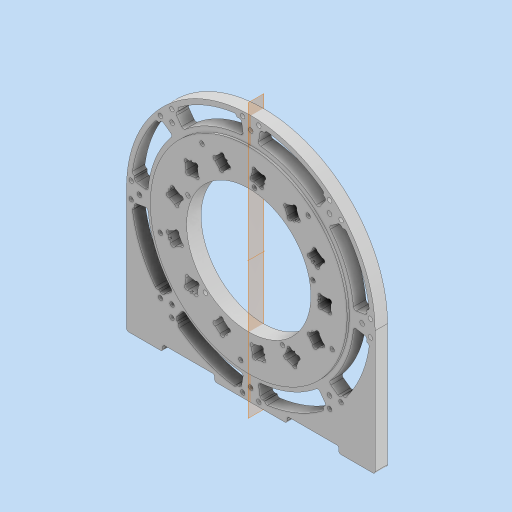
# Autodesk Inventor part: Ring_10_front
Saved by Autodesk Inventor 2024.2 (Build 282272000, 272)
## iProperties
Created: 2025-04-23
Part Number: Ring_10_front
Material: Generic
Document SubType Name: Modeling
Designer: 23661194
Density: 1 g/cm^3
Appearance: Default
Author: 23661194
Autodesk Inventor part; units mm, degrees
ref_plane "XZ Plane" through (0, 0, 0) normal (0, 1, 0) x (-1, 0, 0)
ref_plane "XY Plane" through (0, 0, 0) normal (0, 0, 1) x (1, 0, 0)
sketch "Shim Tray Slot" plane through (0, 0, 0) normal (0, 0, 1) x (1, 0, 0)
  line L0 (30.092, 109.0254) -> (29.9458, 108.3375)
  line L1 (33.5758, 105.3229) -> (31.6829, 97.1237)
  line L2 (-33.5758, 105.3229) -> (-31.6821, 97.1202)
  line L3 (-30.092, 109.0254) -> (-29.9458, 108.3375)
  arc A0 (-32.2001, 107.689) -> (-33.5758, 105.3229) centre (-31.6271, 105.7728) ccw
  arc A1 (29.147, 95.658) -> (-29.1504, 95.657) centre (0, 0) ccw
  arc A2 (28.6337, 111.3782) -> (-28.6337, 111.3782) centre (0, 0) ccw
  arc A3 (-29.9458, 108.3375) -> (-32.2001, 107.689) centre (0, 0) ccw
  arc A4 (32.2001, 107.689) -> (29.9458, 108.3375) centre (0, 0) ccw
  arc A5 (-28.6337, 111.3782) -> (-30.092, 109.0254) centre (-28.1357, 109.4412) ccw
  arc A6 (-31.6821, 97.1202) -> (-29.1504, 95.657) centre (-29.7334, 97.5701) ccw
  arc A7 (29.147, 95.658) -> (31.6829, 97.1237) centre (29.7309, 97.5743) ccw
  arc A8 (33.5758, 105.3229) -> (32.2001, 107.689) centre (31.6271, 105.7728) ccw
  arc A9 (30.092, 109.0254) -> (28.6337, 111.3782) centre (28.1357, 109.4412) ccw
  arc A10 (33.9656, 105.2329) -> (32.3146, 108.0722) centre (31.6271, 105.7728) ccw
  line L4 (33.9656, 105.2329) -> (32.0726, 97.0337)
  arc A11 (29.0304, 95.2754) -> (32.0726, 97.0337) centre (29.7309, 97.5743) ccw
  arc A12 (29.0304, 95.2754) -> (-29.0338, 95.2743) centre (0, 0) ccw
  arc A13 (-32.0718, 97.0302) -> (-29.0338, 95.2743) centre (-29.7334, 97.5701) ccw
  line L5 (-32.0718, 97.0302) -> (-33.9656, 105.2329)
  arc A14 (-32.3146, 108.0722) -> (-33.9656, 105.2329) centre (-31.6271, 105.7728) ccw
  arc A15 (-30.4152, 108.6221) -> (-32.3146, 108.0722) centre (0, 0) ccw
  line L6 (-30.4152, 108.6221) -> (-30.4833, 108.9422)
  arc A16 (-28.7333, 111.7656) -> (-30.4833, 108.9422) centre (-28.1357, 109.4412) ccw
  arc A17 (28.7333, 111.7656) -> (-28.7333, 111.7656) centre (0, 0) ccw
  arc A18 (30.4833, 108.9422) -> (28.7333, 111.7656) centre (28.1357, 109.4412) ccw
  line L7 (30.4833, 108.9422) -> (30.4152, 108.6221)
  arc A19 (32.3146, 108.0722) -> (30.4152, 108.6221) centre (0, 0) ccw
  point P0 (0, 107.5)
  dimension "d188" = 0.4
  measures "d188" radial gap between concentric circles of A2 A17
sketch "Sketch1" plane through (0, 0, 0) normal (0, 0, 1) x (1, 0, 0)
  circle A0 centre (0, 0) radius 60
  circle A1 centre (0, 0) radius 120
  circle A2 centre (0, 0) radius 95
  dimension "d0" = 120
  dimension "d1" = 240
  dimension "d2" = 190
  constraints: 3 centre point, 3 coincident
  measures "d0" diameter of A0
  measures "d1" diameter of A1
  measures "d2" diameter of A2
extrude "Extrusion1" add sketch "Sketch1" along normal blind 12 contours A1 | A2
extrude "Extrusion2" add sketch "Sketch1" along normal blind 14 contours A2
sketch "Sketch2" plane through (0, 0, 14) normal (0, 0, 1) x (1, 0, 0)
  circle A0 centre (0, 0) radius 73.485
  line L0 (73.485, 0) -> (0, 0)
  line L1 (65.0677, 34.1502) -> (0, 0)
  line L2 (41.7442, 60.477) -> (0, 0)
  line L3 (8.8576, 72.9492) -> (0, 0)
  line L4 (-26.0581, 68.7097) -> (0, 0)
  line L5 (-55.0043, 48.7296) -> (0, 0)
  line L6 (-71.3497, 17.5861) -> (0, 0)
  line L7 (-71.3497, -17.5861) -> (0, 0)
  line L8 (-55.0043, -48.7296) -> (0, 0)
  line L9 (-26.0581, -68.7097) -> (0, 0)
  line L10 (8.8576, -72.9492) -> (0, 0)
  line L11 (41.7442, -60.477) -> (0, 0)
  line L12 (65.0677, -34.1502) -> (0, 0)
  line L13 (-168, 0) -> (168, 0) projected
  line L14 (79.425, 5.94) -> (67.545, 5.94)
  line L15 (67.545, 5.94) -> (67.545, -5.94)
  line L16 (67.545, -5.94) -> (79.425, -5.94)
  line L17 (79.425, -5.94) -> (79.425, 5.94)
  line L18 (79.425, 5.94) -> (67.545, -5.94) construction
  line L19 (67.545, 5.94) -> (79.425, -5.94) construction
  circle A1 centre (73.485, 0) radius 2
  circle A2 centre (68.958, -4.527) radius 2.1
  circle A3 centre (78.012, -4.527) radius 2.1
  circle A4 centre (78.012, 4.527) radius 2.1
  circle A5 centre (68.958, 4.527) radius 2.1
  circle A6 centre (67.185, 0) radius 0.75
  line L20 (67.185, 0) -> (73.485, 0)
  line L21 (63.5535, 42.413) -> (56.8049, 32.636)
  line L22 (56.8049, 32.636) -> (66.5819, 25.8874)
  line L23 (66.5819, 25.8874) -> (73.3306, 35.6644)
  line L24 (73.3306, 35.6644) -> (63.5535, 42.413)
  line L25 (63.5535, 42.413) -> (66.5819, 25.8874) construction
  line L26 (56.8049, 32.636) -> (73.3306, 35.6644) construction
  circle A7 centre (65.0677, 34.1502) radius 2
  circle A8 centre (66.2217, 27.8529) radius 2.1
  circle A9 centre (71.365, 35.3042) radius 2.1
  circle A10 centre (63.9137, 40.4475) radius 2.1
  circle A11 centre (58.7705, 32.9962) radius 2.1
  circle A12 centre (61.4889, 28.9654) radius 0.75
  line L27 (61.4889, 28.9654) -> (65.0677, 34.1502)
  line L28 (34.0839, 63.9246) -> (38.2966, 52.8166)
  line L29 (38.2966, 52.8166) -> (49.4046, 57.0293)
  line L30 (49.4046, 57.0293) -> (45.1919, 68.1373)
  line L31 (45.1919, 68.1373) -> (34.0839, 63.9246)
  line L32 (34.0839, 63.9246) -> (49.4046, 57.0293) construction
  line L33 (38.2966, 52.8166) -> (45.1919, 68.1373) construction
  circle A13 centre (41.7442, 60.477) radius 2
  circle A14 centre (47.5824, 57.8494) radius 2.1
  circle A15 centre (44.3718, 66.3151) radius 2.1
  circle A16 centre (35.9061, 63.1045) radius 2.1
  circle A17 centre (39.1167, 54.6389) radius 2.1
  circle A18 centre (43.9782, 54.5864) radius 0.75
  line L34 (43.9782, 54.5864) -> (41.7442, 60.477)
  line L35 (1.6687, 68.6034) -> (13.2035, 65.7603)
  line L36 (13.2035, 65.7603) -> (16.0466, 77.2951)
  line L37 (16.0466, 77.2951) -> (4.5118, 80.1381)
  line L38 (4.5118, 80.1381) -> (1.6687, 68.6034)
  line L39 (1.6687, 68.6034) -> (16.0466, 77.2951) construction
  line L40 (13.2035, 65.7603) -> (4.5118, 80.1381) construction
  circle A19 centre (8.8576, 72.9492) radius 2
  circle A20 centre (14.3365, 76.2613) radius 2.1
  circle A21 centre (5.5456, 78.428) radius 2.1
  circle A22 centre (3.3788, 69.6371) radius 2.1
  circle A23 centre (12.1697, 67.4704) radius 2.1
  circle A24 centre (14.9746, 71.4415) radius 0.75
  line L41 (14.9746, 71.4415) -> (8.8576, 72.9492)
  line L42 (-26.5653, 60.3246) -> (-17.673, 68.2025)
  line L43 (-17.673, 68.2025) -> (-25.5509, 77.0948)
  line L44 (-25.5509, 77.0948) -> (-34.4432, 69.2169)
  line L45 (-34.4432, 69.2169) -> (-26.5653, 60.3246)
  line L46 (-26.5653, 60.3246) -> (-25.5509, 77.0948) construction
  line L47 (-17.673, 68.2025) -> (-34.4432, 69.2169) construction
  circle A25 centre (-26.0581, 68.7097) radius 2
  circle A26 centre (-25.6716, 75.1001) radius 2.1
  circle A27 centre (-32.4486, 69.0962) radius 2.1
  circle A28 centre (-26.4447, 62.3192) radius 2.1
  circle A29 centre (-19.6677, 68.3231) radius 2.1
  circle A30 centre (-21.3425, 72.8873) radius 0.75
  line L48 (-21.3425, 72.8873) -> (-26.0581, 68.7097)
  line L49 (-48.3916, 43.5489) -> (-49.8236, 55.3422)
  line L50 (-49.8236, 55.3422) -> (-61.617, 53.9103)
  line L51 (-61.617, 53.9103) -> (-60.185, 42.1169)
  line L52 (-60.185, 42.1169) -> (-48.3916, 43.5489)
  line L53 (-48.3916, 43.5489) -> (-61.617, 53.9103) construction
  line L54 (-49.8236, 55.3422) -> (-60.185, 42.1169) construction
  circle A31 centre (-55.0043, 48.7296) radius 2
  circle A32 centre (-60.044, 52.6779) radius 2.1
  circle A33 centre (-58.9526, 43.6899) radius 2.1
  circle A34 centre (-49.9646, 44.7812) radius 2.1
  circle A35 centre (-51.056, 53.7692) radius 2.1
  circle A36 centre (-55.7637, 54.9836) radius 0.75
  line L55 (-55.7637, 54.9836) -> (-55.0043, 48.7296)
  line L56 (-63.3296, 20.0853) -> (-73.8488, 25.6062)
  line L57 (-73.8488, 25.6062) -> (-79.3697, 15.087)
  line L58 (-79.3697, 15.087) -> (-68.8505, 9.566)
  line L59 (-68.8505, 9.566) -> (-63.3296, 20.0853)
  line L60 (-63.3296, 20.0853) -> (-79.3697, 15.087) construction
  line L61 (-73.8488, 25.6062) -> (-68.8505, 9.566) construction
  circle A37 centre (-71.3497, 17.5861) radius 2
  circle A38 centre (-77.4619, 15.6815) radius 2.1
  circle A39 centre (-69.445, 11.4739) radius 2.1
  circle A40 centre (-65.2374, 19.4908) radius 2.1
  circle A41 centre (-73.2543, 23.6984) radius 2.1
  circle A42 centre (-76.928, 20.5139) radius 0.75
  line L62 (-76.928, 20.5139) -> (-71.3497, 17.5861)
  line L63 (-68.8505, -9.566) -> (-79.3697, -15.087)
  line L64 (-79.3697, -15.087) -> (-73.8488, -25.6062)
  line L65 (-73.8488, -25.6062) -> (-63.3296, -20.0853)
  line L66 (-63.3296, -20.0853) -> (-68.8505, -9.566)
  line L67 (-68.8505, -9.566) -> (-73.8488, -25.6062) construction
  line L68 (-79.3697, -15.087) -> (-63.3296, -20.0853) construction
  circle A43 centre (-71.3497, -17.5861) radius 2
  circle A44 centre (-73.2543, -23.6984) radius 2.1
  circle A45 centre (-65.2374, -19.4908) radius 2.1
  circle A46 centre (-69.445, -11.4739) radius 2.1
  circle A47 centre (-77.4619, -15.6815) radius 2.1
  circle A48 centre (-76.928, -20.5139) radius 0.75
  line L69 (-76.928, -20.5139) -> (-71.3497, -17.5861)
  line L70 (-60.185, -42.1169) -> (-61.617, -53.9103)
  line L71 (-61.617, -53.9103) -> (-49.8236, -55.3422)
  line L72 (-49.8236, -55.3422) -> (-48.3916, -43.5489)
  line L73 (-48.3916, -43.5489) -> (-60.185, -42.1169)
  line L74 (-60.185, -42.1169) -> (-49.8236, -55.3422) construction
  line L75 (-61.617, -53.9103) -> (-48.3916, -43.5489) construction
  circle A49 centre (-55.0043, -48.7296) radius 2
  circle A50 centre (-51.056, -53.7692) radius 2.1
  circle A51 centre (-49.9646, -44.7812) radius 2.1
  circle A52 centre (-58.9526, -43.6899) radius 2.1
  circle A53 centre (-60.044, -52.6779) radius 2.1
  circle A54 centre (-55.7637, -54.9836) radius 0.75
  line L76 (-55.7637, -54.9836) -> (-55.0043, -48.7296)
  line L77 (-34.4432, -69.2169) -> (-25.5509, -77.0948)
  line L78 (-25.5509, -77.0948) -> (-17.673, -68.2025)
  line L79 (-17.673, -68.2025) -> (-26.5653, -60.3246)
  line L80 (-26.5653, -60.3246) -> (-34.4432, -69.2169)
  line L81 (-34.4432, -69.2169) -> (-17.673, -68.2025) construction
  line L82 (-25.5509, -77.0948) -> (-26.5653, -60.3246) construction
  circle A55 centre (-26.0581, -68.7097) radius 2
  circle A56 centre (-19.6677, -68.3231) radius 2.1
  circle A57 centre (-26.4447, -62.3192) radius 2.1
  circle A58 centre (-32.4486, -69.0962) radius 2.1
  circle A59 centre (-25.6716, -75.1001) radius 2.1
  circle A60 centre (-21.3425, -72.8873) radius 0.75
  line L83 (-21.3425, -72.8873) -> (-26.0581, -68.7097)
  line L84 (4.5118, -80.1381) -> (16.0466, -77.2951)
  line L85 (16.0466, -77.2951) -> (13.2035, -65.7603)
  line L86 (13.2035, -65.7603) -> (1.6687, -68.6034)
  line L87 (1.6687, -68.6034) -> (4.5118, -80.1381)
  line L88 (4.5118, -80.1381) -> (13.2035, -65.7603) construction
  line L89 (16.0466, -77.2951) -> (1.6687, -68.6034) construction
  circle A61 centre (8.8576, -72.9492) radius 2
  circle A62 centre (12.1697, -67.4704) radius 2.1
  circle A63 centre (3.3788, -69.6371) radius 2.1
  circle A64 centre (5.5456, -78.428) radius 2.1
  circle A65 centre (14.3365, -76.2613) radius 2.1
  circle A66 centre (14.9746, -71.4415) radius 0.75
  line L90 (14.9746, -71.4415) -> (8.8576, -72.9492)
  line L91 (45.1919, -68.1373) -> (49.4046, -57.0293)
  line L92 (49.4046, -57.0293) -> (38.2966, -52.8166)
  line L93 (38.2966, -52.8166) -> (34.0839, -63.9246)
  line L94 (34.0839, -63.9246) -> (45.1919, -68.1373)
  line L95 (45.1919, -68.1373) -> (38.2966, -52.8166) construction
  line L96 (49.4046, -57.0293) -> (34.0839, -63.9246) construction
  circle A67 centre (41.7442, -60.477) radius 2
  circle A68 centre (39.1167, -54.6389) radius 2.1
  circle A69 centre (35.9061, -63.1045) radius 2.1
  circle A70 centre (44.3718, -66.3151) radius 2.1
  circle A71 centre (47.5824, -57.8494) radius 2.1
  circle A72 centre (43.9782, -54.5864) radius 0.75
  line L97 (43.9782, -54.5864) -> (41.7442, -60.477)
  line L98 (73.3306, -35.6644) -> (66.582, -25.8874)
  line L99 (66.582, -25.8874) -> (56.8049, -32.636)
  line L100 (56.8049, -32.636) -> (63.5535, -42.413)
  line L101 (63.5535, -42.413) -> (73.3306, -35.6644)
  line L102 (73.3306, -35.6644) -> (56.8049, -32.636) construction
  line L103 (66.582, -25.8874) -> (63.5535, -42.413) construction
  circle A73 centre (65.0677, -34.1502) radius 2
  circle A74 centre (58.7705, -32.9962) radius 2.1
  circle A75 centre (63.9137, -40.4475) radius 2.1
  circle A76 centre (71.365, -35.3042) radius 2.1
  circle A77 centre (66.2218, -27.8529) radius 2.1
  circle A78 centre (61.4889, -28.9654) radius 0.75
  line L104 (61.4889, -28.9654) -> (65.0677, -34.1502)
  point P0 (35.1358, -61.1509)
  point P1 (36.8576, -64.9766)
  point P2 (42.4181, -67.0854)
  point P3 (46.2438, -65.3636)
  point P4 (48.3526, -59.8031)
  point P5 (46.6308, -55.9774)
  point P6 (41.0703, -53.8686)
  point P7 (37.2447, -55.5904)
  point P8 (4.549, -67.8934)
  point P9 (2.3786, -71.4837)
  point P10 (3.8018, -77.2578)
  point P11 (7.3921, -79.4282)
  point P12 (13.1662, -78.005)
  point P13 (15.3366, -74.4148)
  point P14 (13.9134, -68.6406)
  point P15 (10.3232, -66.4702)
  point P16 (-24.3449, -62.2917)
  point P17 (-28.5325, -62.545)
  point P18 (-32.4761, -66.9964)
  point P19 (-32.2228, -71.184)
  point P20 (-27.7714, -75.1276)
  point P21 (-23.5838, -74.8743)
  point P22 (-19.6402, -70.4229)
  point P23 (-19.8935, -66.2353)
  point P24 (-49.466, -52.3974)
  point P25 (-48.7492, -46.4938)
  point P26 (-51.3365, -43.1913)
  point P27 (-57.2401, -42.4745)
  point P28 (-60.5426, -45.0618)
  point P29 (-61.2594, -50.9654)
  point P30 (-58.6721, -54.2678)
  point P31 (-52.7685, -54.9847)
  point P32 (-67.4719, -12.1928)
  point P33 (-71.4772, -10.9447)
  point P34 (-76.743, -13.7083)
  point P35 (-77.9911, -17.7137)
  point P36 (-75.2274, -22.9795)
  point P37 (-71.2221, -24.2276)
  point P38 (-65.9563, -21.4639)
  point P39 (-64.7082, -17.4585)
  point P40 (-64.7082, 17.4585)
  point P41 (-65.9563, 21.4639)
  point P42 (-71.2221, 24.2276)
  point P43 (-75.2274, 22.9795)
  point P44 (-77.9911, 17.7137)
  point P45 (-76.743, 13.7083)
  point P46 (-71.4772, 10.9447)
  point P47 (-67.4719, 12.1928)
  point P48 (-51.3365, 43.1913)
  point P49 (-48.7492, 46.4938)
  point P50 (-49.466, 52.3974)
  point P51 (-52.7685, 54.9847)
  point P52 (-58.6721, 54.2678)
  point P53 (-61.2594, 50.9654)
  point P54 (-60.5426, 45.0618)
  point P55 (-57.2401, 42.4745)
  point P56 (-19.8935, 66.2353)
  point P57 (-19.6402, 70.4229)
  point P58 (-23.5838, 74.8743)
  point P59 (-27.7714, 75.1276)
  point P60 (-32.2228, 71.184)
  point P61 (-32.4761, 66.9964)
  point P62 (-28.5325, 62.545)
  point P63 (-24.3449, 62.2917)
  point P64 (2.3786, 71.4837)
  point P65 (4.549, 67.8934)
  point P66 (10.3232, 66.4702)
  point P67 (13.9134, 68.6406)
  point P68 (15.3366, 74.4148)
  point P69 (13.1662, 78.005)
  point P70 (7.3921, 79.4282)
  point P71 (3.8018, 77.2578)
  point P72 (48.3526, 59.8031)
  point P73 (46.2438, 65.3636)
  point P74 (42.4181, 67.0854)
  point P75 (36.8576, 64.9766)
  point P76 (35.1358, 61.1509)
  point P77 (37.2447, 55.5904)
  point P78 (41.0703, 53.8686)
  point P79 (46.6308, 55.9774)
  point P80 (68.2671, 28.3287)
  point P81 (71.6454, 33.223)
  point P82 (70.8892, 37.3496)
  point P83 (65.9949, 40.7278)
  point P84 (61.8683, 39.9716)
  point P85 (58.4901, 35.0774)
  point P86 (59.2463, 30.9508)
  point P87 (64.1405, 27.5725)
  point P88 (79.425, 2.9735)
  point P89 (76.4585, 5.94)
  point P90 (70.5115, 5.94)
  point P91 (67.545, 2.9735)
  point P92 (67.545, -2.9735)
  point P93 (70.5115, -5.94)
  point P94 (76.4585, -5.94)
  point P95 (79.425, -2.9735)
  point P96 (58.4901, -35.0774)
  point P97 (61.8683, -39.9716)
  point P98 (65.9949, -40.7278)
  point P99 (70.8892, -37.3496)
  point P100 (71.6454, -33.223)
  point P101 (68.2671, -28.3288)
  point P102 (64.1406, -27.5725)
  point P103 (59.2463, -30.9508)
  dimension "d7" = 146.97
  dimension "d123" = -55.385
  dimension "d124" = -110.769
  dimension "d125" = -166.154
  dimension "d126" = -221.538
  dimension "d127" = -276.923
  dimension "d129" = -27.692
  dimension "d130" = -83.077
  dimension "d131" = -138.462
  dimension "d132" = -193.846
  dimension "d133" = -249.231
  dimension "d134" = -304.615
  dimension "d120" = 360
  dimension "d122" = 0
  dimension "d128" = -332.308
  constraints: 26 end point, 2 horizontal, 1 coincident, 1 horizontal alignment, 56 other
  measures "d122" vertical extent of L0
extrude "Extrusion3" cut sketch "Sketch2" against normal blind 12 contours L0 A1 A0 | L13 A1 A0 | A0 A1 L0 | A0 A1 L13 | A1 L0 A6 L15 A5 L14 A0 | A0 L14 A4 L17 L13 A1 | A1 L13 L17 A3 L16 A0 | A0 L16 A2 L15 A6 L0 A1 | A6 L15 L0 | L0 L15 A6 | A8 L22 L23 A0 | A0 L23 A8 | A4 L17 L14 | L14 L17 A4 | A5 L15 L14 | L14 L15 A5 | A77 L98 A0 | A0 L98 L99 A77 | A2 L15 L16 | L16 L15 A2 | A3 L17 L16 | L16 L17 A3 | L23 L22 A8 A0 | A0 A8 L23 | L22 A12 L27 A7 A0 A8 | L98 A77 A0 | A0 A77 L99 L98 | A77 A0 A73 L104 A78 L99 | A0 A7 L21 A10 L24 A9 L23 A8 | L22 L27 A12 | A77 L98 A76 L101 A75 L100 A0 A73 | A78 L104 L99 | A7 L27 A0 | A0 A7 | A9 L24 L23 | L23 L24 A9 | L22 A12 L27 | L22 A11 L1 A7 L27 A12 | A73 A0 | A0 L104 A73 | A76 L101 L98 | L98 L101 A76 | L104 A78 L99 | A78 L104 A73 L12 A74 L99 | A11 L21 L22 L1 | L1 L22 A11 | A17 L28 L2 | L2 L28 L29 A17 | L35 A22 L38 A0 A19 L3 | L3 A19 L41 A24 L36 A23 L35 | L42 A28 L45 A0 A25 L4 | L4 A25 A0 L43 A29 L42 | A34 L52 L5 | L5 L52 L49 A34 | L59 A39 L58 A0 A37 L6 | L6 A37 A0 L56 A40 L59 | L66 A45 L65 A0 A43 L7 | L7 A43 A0 L63 A46 L66 | A51 L72 L73 L8 | L8 L73 A51 | L79 A56 L78 A0 A55 L9 | L9 A55 A0 L80 A57 L79 | L86 A62 L85 A66 L90 A61 L10 | L10 A61 A0 L87 A63 L86 | A68 L92 L93 L11 | L11 L93 A68 | A74 L99 L12 | L12 L99 L100 A74 | L1 A7 A0 | L27 A7 L1 | L22 L1 A11 | A0 A73 L12 | L12 A73 L104 | A74 L12 L99 | L22 L21 A11 L1 | L21 A0 A7 L1 A11 | L28 A17 L2 | L2 A17 L29 L28 | L28 A16 A0 A13 L2 A17 | A17 L2 A13 L34 A18 L29 | A19 A0 L3 | L3 L41 A19 | A22 L38 L35 | L35 L38 A22 | A23 L36 L35 | L35 L36 A23 | A25 A0 L4 | L4 A0 A25 | A28 L45 L42 | L42 L45 A28 | A29 L43 L42 | L42 L43 A29 | L52 A34 L5 | L5 A34 L49 L52 | L52 A33 A0 A31 L5 A34 | A37 A0 L6 | L6 A0 A37 | A39 L58 L59 | L59 L58 A39 | A40 L56 L59 | L59 L56 A40 | A43 A0 L7 | L7 A0 A43 | A45 L65 L66 | L66 L65 A45 | A46 L63 L66 | L66 L63 A46 | L73 L72 A51 L8 | L8 A51 L73 | A51 L8 A49 A0 A52 L73 | A55 A0 L9 | L9 A0 A55 | A56 L78 L79 | L79 L78 A56 | A57 L80 L79 | L79 L80 A57 | A61 L90 L10 | L10 A0 A61 | A62 L85 L86 | L86 L85 A62 | A63 L87 L86 | L86 L87 A63 | L93 L92 A68 L11 | L11 A68 L93 | L92 A72 L97 A67 L11 A68 | A68 L11 A67 A0 A69 L93 | L12 A74 L100 L99 | A74 L12 A73 A0 L100 | L58 A38 L57 A42 L62 A37 A0 | A0 A43 L69 A48 L64 A47 L63 | A10 L21 L24 | L24 L21 A10 | A75 L100 L101 | L101 L100 A75 | A16 A0 L31 L28 | L28 L31 A0 A16 | A18 L34 L29 | A0 A19 | A0 A19 L41 | A0 L38 A21 L37 A20 L36 A24 A19 | A19 A0 A24 L41 | L48 A25 A0 | A0 A25 L48 | A0 L45 A27 L44 A26 L43 A30 L48 A25 | L5 A31 A0 A35 L49 A34 | A33 A0 L51 L52 | L52 L51 A0 A33 | L62 A37 A0 | A0 A37 L62 | L69 A43 A0 | A0 A43 L69 | A51 L72 A50 A0 A49 L8 | A52 A0 L70 L73 | L73 L70 A0 A52 | L83 A55 A0 | A0 A55 L83 | A55 L83 A60 L78 A59 L77 A58 L80 A0 | A0 A61 | L90 A61 A0 | L90 A66 A0 A61 | A61 A0 A66 L85 A65 L84 A64 L87 | L92 L97 A72 | A69 A0 L94 L93 | L93 L94 A0 A69 | A38 L57 L58 | L58 L57 A38 | A47 L64 L63 | L63 L64 A47 | A14 L29 A0 | A0 L29 L30 A14 | A13 A0 L2 | L2 L34 A13 | A16 L31 A0 | A16 L31 A15 L30 A14 A0 A13 | A0 L31 A16 | L34 A18 L29 | L34 A13 A0 A14 L29 A18 | L41 L36 A24 | A24 A0 L36 L41 | A25 L48 A30 L43 A0 | A31 A0 L5 | L5 A0 A31 | A33 L51 A0 | A35 A0 L49 | L49 A0 A35 | A37 L62 A42 L57 A41 L56 A0 | A0 L65 A44 L64 A48 L69 A43 | A49 A0 L8 | L8 A0 A49 | A50 A0 L72 | L72 A0 A50 | A0 L70 A52 | A0 L78 A60 L83 A55 | L90 L85 A0 A66 | A66 L85 L90 | A67 L97 L11 | L11 A0 A67 | L92 A72 L97 | A72 L92 A71 A0 A67 L97 | A69 L94 A0 | A0 A67 A71 L91 A70 L94 A69 | A0 L94 A69 | A71 L91 L92 A0 | A0 L92 A71 | L29 A14 A0 | A0 A14 L30 L29 | A0 A13 | A0 A13 L34 | A24 L36 A0 | A21 L37 L38 | L38 L37 A21 | L48 L43 A30 | A30 L43 L48 | A0 L49 L50 A35 | A27 L44 L45 | L45 L44 A27 | L55 A31 A0 | A0 A31 L55 | A0 A33 L51 A32 L50 A36 L55 A31 | L51 A33 A0 | A0 A35 L50 L49 | A0 A31 L55 A36 L50 A35 | L62 L57 A42 | A42 L57 L62 | A41 L57 L56 | L56 L57 A41 | L69 L64 A48 | A48 L64 L69 | A44 L64 L65 | L65 L64 A44 | L76 A49 A0 | A0 A49 L76 | A49 L76 A54 L71 A53 L70 A52 A0 | L72 L71 A50 A0 | A0 A50 L71 L72 | A50 L71 A54 L76 A49 A0 | A0 A52 L70 | L83 L78 A60 | A60 L78 L83 | A58 L77 L80 | L80 L77 A58 | A0 L85 A66 | A64 L84 L87 | L87 L84 A64 | A0 A67 | L97 A67 A0 | L92 L91 A71 A0 | A0 A71 L92 | A15 L30 L31 | L31 L30 A15 | A32 L50 L51 | L51 L50 A32 | A53 L71 L70 | L70 L71 A53 | A70 L91 L94 | L94 L91 A70 | A20 L37 L36 | L36 L37 A20 | A26 L44 L43 | L43 L44 A26 | A36 L55 L50 | A36 L50 L55 | L76 L71 A54 | A54 L71 L76 | A59 L77 L78 | L78 L77 A59 | A65 L84 L85 | L85 L84 A65 picked at (67.5888, -0.4081) picked at (67.5888, 0.4081) picked at (14.7369, 72.0977) picked at (14.7369, -72.0977)
extrude "Extrusion4" cut sketch "Sketch2" against normal blind 2 contours A6 L15 L0 | L0 L15 A6 | L15 A6 L0 | L0 A6 L15 | A12 L22 | L22 L27 A12 | A78 L104 L99 | L99 A78 | L22 A12 L27 | L104 A78 L99 | A18 L34 L29 | L29 A18 | A72 L92 | L92 L97 A72 | L34 A18 L29 | L41 L36 A24 | A24 A0 L36 L41 | L36 A0 A24 | L90 L85 A0 A66 | A66 L85 L90 | A66 A0 L85 | L92 A72 L97 | A0 L36 A24 | A24 L36 A0 | L48 L43 A30 | A30 L43 L48 | L43 A30 | L62 L57 A42 | A42 L57 L62 | L69 L64 A48 | A48 L64 L69 | L83 L78 A60 | A60 L78 L83 | A60 L78 | A0 L85 A66 | A66 L85 A0 | A42 L57 | L64 A48 | A36 L55 L50 | L50 A36 | A36 L50 L55 | L76 L71 A54 | A54 L71 L76 | A54 L71
extrude "Extrusion5" cut sketch "Sketch2" against normal through all contours L0 A1 A0 | L13 A1 A0 | A0 A1 L0 | A0 A1 L13 | A7 L27 A0 | A0 A7 | A73 A0 | A0 L104 A73 | L1 A7 A0 | L27 A7 L1 | A0 A73 L12 | L12 A73 L104 | A19 A0 L3 | L3 L41 A19 | A25 A0 L4 | L4 A0 A25 | A37 A0 L6 | L6 A0 A37 | A43 A0 L7 | L7 A0 A43 | A55 A0 L9 | L9 A0 A55 | A61 L90 L10 | L10 A0 A61 | A0 A19 | A0 A19 L41 | L48 A25 A0 | A0 A25 L48 | L62 A37 A0 | A0 A37 L62 | L69 A43 A0 | A0 A43 L69 | L83 A55 A0 | A0 A55 L83 | A0 A61 | L90 A61 A0 | A13 A0 L2 | L2 L34 A13 | A31 A0 L5 | L5 A0 A31 | A49 A0 L8 | L8 A0 A49 | A67 L97 L11 | L11 A0 A67 | A0 A13 | A0 A13 L34 | L55 A31 A0 | A0 A31 L55 | L76 A49 A0 | A0 A49 L76 | A0 A67 | L97 A67 A0
sketch "Sketch3" plane through (0, 0, 12) normal (0, 0, 1) x (1, 0, 0)
  circle A0 centre (0, 0) radius 107.5
  circle A1 centre (0, 107.5) radius 2.15
  circle A2 centre (-76.014, 76.014) radius 2.15
  circle A3 centre (-107.5, 0) radius 2.15
  circle A4 centre (-76.014, -76.014) radius 2.15
  circle A5 centre (0, -107.5) radius 2.15
  circle A6 centre (76.014, -76.014) radius 2.15
  circle A7 centre (107.5, 0) radius 2.15
  circle A8 centre (76.014, 76.014) radius 2.15
  dimension "d141" = 215
  dimension "d142" = 4.3
  dimension "d145" = 360
  constraints: 8 centre point, 1 coincident, 1 vertical alignment, 19 other
  measures "d142" diameter of A1
extrude "Extrusion6" cut sketch "Sketch3" against normal through all contours A0 A7 | A0 A7 | A8 A0 | A0 A8 | A6 A0 | A0 A6 | A1 A0 | A0 A1 | A5 A0 | A0 A5 | A2 A0 | A0 A2 | A4 A0 | A0 A4 | A3 A0 | A0 A3
sketch "Sketch4" plane through (0, 0, 14) normal (0, 0, 1) x (1, 0, 0)
  circle A0 centre (0, 0) radius 63.75
  line L0 (0, 0) -> (5.5562, 63.5074)
  circle A1 centre (5.5562, 63.5074) radius 2.1
  line L1 (0, 168) -> (0, -168) projected
  circle A2 centre (-58.6822, 24.9091) radius 2.1
  circle A3 centre (-41.8238, -48.1127) radius 2.1
  circle A4 centre (32.8337, -54.6444) radius 2.1
  circle A5 centre (62.1161, 14.3406) radius 2.1
  circle A6 centre (0, 0) radius 87.5
  line L2 (0, 0) -> (57.4052, 66.0371)
  circle A7 centre (57.4052, 66.0371) radius 2.1
  circle A8 centre (-45.0658, 75.0021) radius 2.1
  circle A9 centre (-85.2574, -19.6832) radius 2.1
  circle A10 centre (-7.6261, -87.167) radius 2.1
  circle A11 centre (80.5442, -34.189) radius 2.1
  dimension "d149" = 127.5
  dimension "d156" = 175
  dimension "d150" = 4.2
  dimension "d151" = 5
  dimension "d154" = 360
  dimension "d157" = 4.2
  dimension "d158" = 41
  dimension "d161" = 360
  constraints: 10 centre point, 5 coincident, 4 end point, 1 midpoint, 28 other
  measures "d150" diameter of A1
  measures "d151" angle of L1 L0
  measures "d157" diameter of A7
  measures "d158" angle of L1 L2
extrude "Extrusion7" cut sketch "Sketch4" against normal blind 8 contours A5 A0 | A0 A5 | A4 A0 | A0 A4 | A1 L0 A0 | A0 A1 | A7 A6 L2 | L2 A6 A7 | A3 A0 | A0 A3 | L0 A1 A0 | A6 A7 | A10 A6 | A6 A10 | A11 A6 | A6 A11 | A2 A0 | A0 A2 | A8 A6 | A6 A8 | A9 A6 | A6 A9
sketch "Sketch5" plane through (0, 0, 12) normal (0, 0, 1) x (1, 0, 0)
  circle A0 centre (0, 0) radius 120 projected
  line L0 (-120, 0) -> (-120, -120)
  line L1 (-120, -120) -> (120, -120)
  line L2 (120, -120) -> (120, 0)
  line L3 (-35, -114) -> (-85, -114)
  line L4 (-85, -114) -> (-85, -126)
  line L5 (-85, -126) -> (-35, -126)
  line L6 (-35, -126) -> (-35, -114)
  line L7 (-35, -114) -> (-85, -126) construction
  line L8 (-85, -114) -> (-35, -126) construction
  line L9 (85, -114) -> (35, -114)
  line L10 (35, -114) -> (35, -126)
  line L11 (35, -126) -> (85, -126)
  line L12 (85, -126) -> (85, -114)
  line L13 (85, -114) -> (35, -126) construction
  line L14 (35, -114) -> (85, -126) construction
  point P0 (-60, -120)
  point P1 (60, -120)
  point P2 (37.47, -114)
  point P3 (85, -120)
  point P4 (35, -120)
  point P5 (35, -114.7824)
  point P6 (0, -120)
  point P7 (-35, -114.7824)
  point P8 (-35, -120)
  point P9 (-85, -120)
  point P10 (-37.47, -114)
  dimension "d165" = 120
  dimension "d166" = 240
  dimension "d167" = 60
  dimension "d168" = 60
  dimension "d169" = 50
  dimension "d170" = 50
  dimension "d171" = 12
  constraints: 30 end point, 4 midpoint, 4 parallel, 4 perpendicular, 3 point on line, 2 horizontal, 2 point on circle, 1 tangent, 1 vertical
  measures "d165" distance of L0.start L0.end
  measures "d166" distance of L0.end L1.end
  measures "d167" distance from line of L0 point (-60, -120)
  measures "d168" distance from line of L2 point (60, -120)
  measures "d169" distance of L5.end L4.end
  measures "d170" distance of L11.end L10.end
  measures "d171" distance between parallel lines of L5 L3
extrude "Extrusion8" add sketch "Sketch5" against normal blind 12 contours L2 L1 L12 L9 A0 | A0 L3 L4 L1 L0 | L10 L1 A0 | A0 L1 L6
extrude "Extrusion9" cut sketch "Sketch5" against normal blind 12 contours A0 L10 L9 | L3 L6 A0
fillet "Fillet1" radius 2 10 edges at (-120, -120, 6) (-85, -120, 6) (-85, -114, 6) (-35, -114, 6) (-35, -120, 6) (35, -114, 6) (35, -120, 6) (85, -114, 6) (85, -120, 6) (120, -120, 6)
sketch "Sketch7" plane through (0, 0, 12) normal (0, 0, 1) x (1, 0, 0)
  circle A0 centre (0, 107.5) radius 2.15 projected
  circle A1 centre (0, 0) radius 107.5
  line L0 (0, 0) -> (41.1385, 99.317)
  line L1 (0, 168) -> (0, -168) projected
  circle A2 centre (0, 0) radius 115.75
  circle A3 centre (7.7881, 115.4877) radius 2.1
  circle A4 centre (76.1551, 87.1691) radius 2.1
  line L2 (69.5236, 89.2106) -> (69.1253, 88.631)
  line L3 (71.3254, 84.4568) -> (66.4388, 77.6061)
  line L4 (9.2853, 110.1546) -> (7.8959, 101.8516)
  line L5 (13.9208, 112.2421) -> (13.7927, 111.5505)
  arc A5 (11.4618, 111.8141) -> (9.2853, 110.1546) centre (11.2579, 109.8245) ccw
  arc A6 (63.5351, 77.2224) -> (9.6749, 99.5309) centre (0, 0) ccw
  arc A7 (69.0767, 91.9424) -> (16.1685, 113.8577) centre (0, 0) ccw
  arc A8 (13.7927, 111.5505) -> (11.4618, 111.8141) centre (0, 0) ccw
  arc A9 (70.9598, 87.1692) -> (69.1253, 88.631) centre (0, 0) ccw
  arc A10 (16.1685, 113.8577) -> (13.9208, 112.2421) centre (15.8873, 111.8776) ccw
  arc A11 (7.8959, 101.8516) -> (9.6749, 99.5309) centre (9.8684, 101.5215) ccw
  arc A12 (63.5351, 77.2224) -> (66.4388, 77.6061) centre (64.8079, 78.7694) ccw
  arc A13 (71.3254, 84.4568) -> (70.9598, 87.1692) centre (69.6971, 85.6182) ccw
  arc A14 (69.5236, 89.2106) -> (69.0767, 91.9424) centre (67.8754, 90.3434) ccw
  arc A15 (71.651, 84.2245) -> (71.2123, 87.4794) centre (69.6971, 85.6182) ccw
  line L6 (71.651, 84.2245) -> (66.7645, 77.3738)
  arc A16 (63.2809, 76.9135) -> (66.7645, 77.3738) centre (64.8079, 78.7694) ccw
  arc A17 (63.2809, 76.9135) -> (9.6362, 99.1328) centre (0, 0) ccw
  arc A18 (7.5013, 101.9176) -> (9.6362, 99.1328) centre (9.8684, 101.5215) ccw
  line L7 (7.5013, 101.9176) -> (8.8908, 110.2206)
  arc A19 (11.5026, 112.212) -> (8.8908, 110.2206) centre (11.2579, 109.8245) ccw
  arc A20 (13.4679, 111.9931) -> (11.5026, 112.212) centre (0, 0) ccw
  line L8 (13.4679, 111.9931) -> (13.5275, 112.3149)
  arc A21 (16.2248, 114.2537) -> (13.5275, 112.3149) centre (15.8873, 111.8776) ccw
  arc A22 (69.317, 92.2622) -> (16.2248, 114.2537) centre (0, 0) ccw
  arc A23 (69.8533, 88.9841) -> (69.317, 92.2622) centre (67.8754, 90.3434) ccw
  line L9 (69.8533, 88.9841) -> (69.6679, 88.7143)
  arc A24 (71.2123, 87.4794) -> (69.6679, 88.7143) centre (0, 0) ccw
  point P0 (70.9598, 87.1692)
  point P1 (71.2123, 87.4794)
  dimension "d180" = 22.5
  dimension "d194" = 231.5
  dimension "d195" = 4.2
  dimension "d199" = 4.2
  dimension "d201" = 37
  dimension "d202" = 37
  constraints: 4 centre point, 4 point on circle, 3 coincident, 2 end point, 3 other
  measures "d180" angle of L1 L0
  measures "d194" diameter of A2
  measures "d195" diameter of A3
  measures "d199" diameter of A4
  measures "d201" distance from line of A3.centre L0
  measures "d202" distance from line of A4.centre L0
extrude "Extrusion12" cut sketch "Sketch7" against normal through all contours L7 A19 A20 L8 A21 A22 A23 L9 A24 A15 L6 A1 L3 A13 A9 L2 A14 A7 A10 L5 A8 A5 L4 | A1 L4 A11 A6 L0 A17 A18 L7 | L4 A5 A8 L5 A10 A7 A14 L2 A9 A13 L3 A1 | A1 L0 A6 A11 L4 | L0 A6 A12 L3 A1 L6 A16 A17 | A1 L3 A12 A6 L0
pattern_circular "Circular Pattern2" count 8 over 360 about axis through (0, 0, -10) along (0, 0, 1) of "Extrusion12"
extrude "Extrusion13" cut sketch "Sketch7" against normal blind 8 contours A3 A2 | A2 A3 | A4 A2 | A2 A4
pattern_circular "Circular Pattern3" count 8 over 360 about axis through (0, 0, -10) along (0, 0, 1) of "Extrusion13"
sketch "Block2" plane through (0, 0, 0) normal (0, 0, 1) x (1, 0, 0)
  line L0 (83.1381, 5.88) -> (71.258, 5.88)
  line L1 (71.258, 5.88) -> (71.258, -6)
  line L2 (71.258, -6) -> (83.1381, -6)
  line L3 (83.1381, -6) -> (83.1381, 5.88)
  line L4 (83.1381, 5.88) -> (71.258, -6) construction
  line L5 (71.258, 5.88) -> (83.1381, -6) construction
  circle A0 centre (77.198, -0.06) radius 2
  circle A1 centre (72.671, -4.587) radius 2.1
  circle A2 centre (81.725, -4.587) radius 2.1
  circle A3 centre (81.725, 4.467) radius 2.1
  circle A4 centre (72.671, 4.467) radius 2.1
  circle A5 centre (70.898, -0.06) radius 0.75
  line L6 (70.898, -0.06) -> (77.198, -0.06)
  dimension "d13" = 11.88
  dimension "d15" = 4.2
  dimension "d12" = 11.88
  dimension "d14" = 4
  dimension "d16" = 1.413
  dimension "d17" = 360
  dimension "d18" = 1.5
  dimension "d19" = 6.3
  constraints: 6 end point, 2 centre point, 2 coincident, 2 midpoint, 1 horizontal, 1 point on line, 21 other
  measures "d12" distance of L5.end L4.end
  measures "d14" diameter of A0
  measures "d18" diameter of A5
  measures "d19" distance of L6.end L6.start
body "Solid1"
